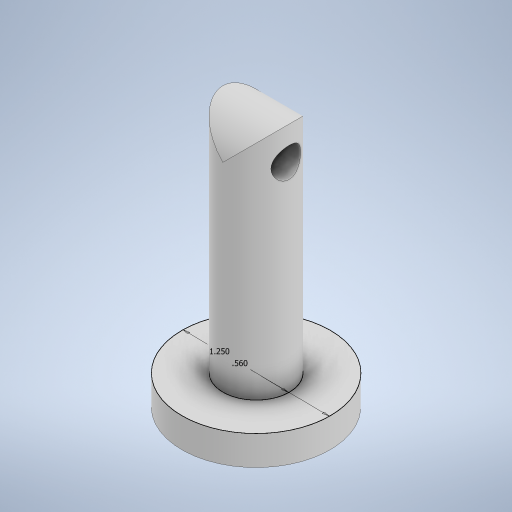
# Autodesk Inventor part: Load Cell Test Mount to Find Required Torque Application
Saved by Autodesk Inventor 2023 (Build 270158000, 158)
## iProperties
Created: 2023-02-15
Part Number: Load Cell Test Mount to Find Required Torque Application
Material: Generic
Document SubType Name: Modeling
Designer: tommy
Density: 1 g/cm^3
Appearance: Default
Author: tommy
Autodesk Inventor part; units mm, degrees
ref_plane "YZ Plane" through (0, 0, 0) normal (1, 0, 0) x (0, 1, 0)
ref_plane "XZ Plane" through (0, 0, 0) normal (0, 1, 0) x (-1, 0, 0)
ref_plane "XY Plane" through (0, 0, 0) normal (0, 0, 1) x (1, 0, 0)
sketch "Sketch1" plane through (0, 0, 0) normal (0, 1, 0) x (-1, 0, 0)
  circle A0 centre (0, 0) radius 15.875
  circle A1 centre (0, 0) radius 7.112
  dimension "d0" = 31.75
  dimension "d1" = 14.224
  constraints: 2 centre point, 2 coincident
  measures "d0" diameter of A0
  measures "d1" diameter of A1
extrude "Extrusion1" add sketch "Sketch1" along normal blind 50.8 contours A1
extrude "Extrusion2" add sketch "Sketch1" against normal blind 6.35 contours A0 | A1
sketch "Sketch2" plane through (0, 0, 0) normal (1, 0, 0) x (0, 1, 0)
  line L0 (50.8, -7.112) -> (50.8, 7.112) projected
  circle A0 centre (42.6249, 0) radius 3.175
  circle A1 centre (42.6249, 0) radius 7.112
  line L1 (0, -7.112) -> (50.8, -7.112) projected
  line L2 (42.6249, -7.112) -> (42.6249, -13.9262)
  line L3 (42.6249, -13.9262) -> (57.419, -13.9262)
  line L4 (57.419, -13.9262) -> (57.419, 14.0929)
  line L5 (57.419, 14.0929) -> (42.6249, 14.0929)
  line L6 (42.6249, 14.0929) -> (42.6249, 7.112)
  point P0 (0, 0)
  point P1 (39.4499, 0)
  dimension "d7" = 6.35
  constraints: 10 end point, 3 perpendicular, 2 point on circle, 2 point on line, 1 centre point, 1 coincident, 1 horizontal alignment, 1 vertical, 2 other
extrude "Extrusion3" cut sketch "Sketch2" along normal mid plane 127 contours A0 | A1 L6 L5 L4 L3 L2
body "Solid1"
